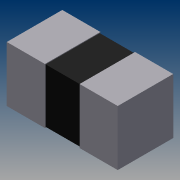
# Autodesk Inventor part: 0603
Saved by Autodesk Inventor 2011 (Build 150239000, 239)
## iProperties
Created: 2010-10-15
Part Number: 0603
Document SubType Name: Modeling
Designer: abbath
Density: 1 g/cm^3
Mass: 0.0010082 g
Surface Area: 0.064232 cm^2
Volume: 0.0010082 cm^3
Author: abbath
Autodesk Inventor part; units mm, degrees
ref_plane "YZ Plane" through (0, 0, 0) normal (1, 0, 0) x (0, 1, 0)
ref_plane "XZ Plane" through (0, 0, 0) normal (0, 1, 0) x (-1, 0, 0)
ref_plane "XY Plane" through (0, 0, 0) normal (0, 0, 1) x (1, 0, 0)
sketch "Эскиз1" plane through (0, 0, 0) normal (0, 0, 1) x (1, 0, 0)
  line L0 (-0.8, 0.4) -> (0.8, 0.4)
  line L1 (0.8, 0.4) -> (0.8, -0.4)
  line L2 (0.8, -0.4) -> (-0.8, -0.4)
  line L3 (-0.8, -0.4) -> (-0.8, 0.4)
  point P0 (0, 0)
  dimension "d0" = 1.6
  dimension "d1" = 0.8
  dimension "d2" = 0.8
  dimension "d3" = 0.8
  dimension "d4" = 0.4
  dimension "d5" = 0.4
  constraints: 8 end point, 2 parallel, 1 horizontal, 1 perpendicular
  measures "d0" distance between parallel lines of L1 L3
  measures "d1" distance between parallel lines of L2 L0
  measures "d2" distance from line of L3 point (0, 0)
  measures "d3" distance from line of L1 point (0, 0)
  measures "d4" distance from line of L2 point (0, 0)
  measures "d5" distance from line of L0 point (0, 0)
extrude "Выдавливание1" add sketch "Эскиз1" along normal blind 0.8
sketch "Эскиз2" plane through (0, 0, 0.8) normal (0, 0, 1) x (1, 0, 0)
  line L0 (0.8, 0.4) -> (0.8, -0.4) projected
  line L1 (-0.8, 0.4) -> (0.8, 0.4) projected
  line L2 (-0.8, -0.4) -> (-0.8, 0.4) projected
  line L3 (0.8, -0.4) -> (-0.8, -0.4) projected
  line L4 (-0.25, 0.4) -> (-0.25, -0.4)
  line L5 (0.25, 0.4) -> (0.25, -0.4)
  point P0 (0, 0)
  dimension "d10" = 0.5
  dimension "d11" = 0.55
  dimension "d12" = 0.55
  constraints: 4 end point, 4 point on line, 2 perpendicular
  measures "d10" distance between parallel lines of L5 L4
  measures "d11" distance between parallel lines of L4 L2
  measures "d12" distance between parallel lines of L0 L5
extrude "Выдавливание2" cut sketch "Эскиз2" against normal blind 0.01 contours L5 L3 L4 L1
sketch "Эскиз3" plane through (-0.8, -0.4, 0) normal (0, -1, 0) x (1, 0, 0)
  line L0 (1.6, 0) -> (0, 0) projected
  line L1 (1.05, 0.79) -> (0.55, 0.79) projected
  line L2 (0.55, 0.79) -> (0.55, 0)
  line L3 (1.05, 0.79) -> (1.05, 0)
  point P0 (0.8, 0)
  constraints: 4 end point, 2 perpendicular, 2 point on line
extrude "Выдавливание3" cut sketch "Эскиз3" against normal blind 0.01
sketch "Эскиз4" plane through (0, 0, 0) normal (0, 0, -1) x (-1, 0, 0)
  line L0 (-0.25, -0.39) -> (0.25, -0.39) projected
  line L1 (0.8, 0.4) -> (-0.8, 0.4) projected
  line L2 (0.25, -0.39) -> (0.25, 0.4)
  line L3 (-0.25, -0.39) -> (-0.25, 0.4)
  point P0 (0, 0)
  constraints: 4 end point, 2 perpendicular, 2 point on line
extrude "Выдавливание4" cut sketch "Эскиз4" against normal blind 0.01
sketch "Эскиз5" plane through (-0.8, 0.4, 0.8) normal (0, 1, 0) x (1, 0, 0)
  line L0 (0.55, 0.01) -> (1.05, 0.01) projected
  line L1 (1.05, 0.79) -> (0.55, 0.79) projected
  line L2 (0.55, 0.79) -> (0.55, 0.01)
  line L3 (1.05, 0.79) -> (1.05, 0.01)
  point P0 (0.8, 0.8)
  constraints: 4 end point, 1 parallel, 1 perpendicular
extrude "Выдавливание5" cut sketch "Эскиз5" against normal blind 0.01
equation "\"d2\" = d3"
equation "\"d4\" = d5"
equation "\"d11\" = d12"
